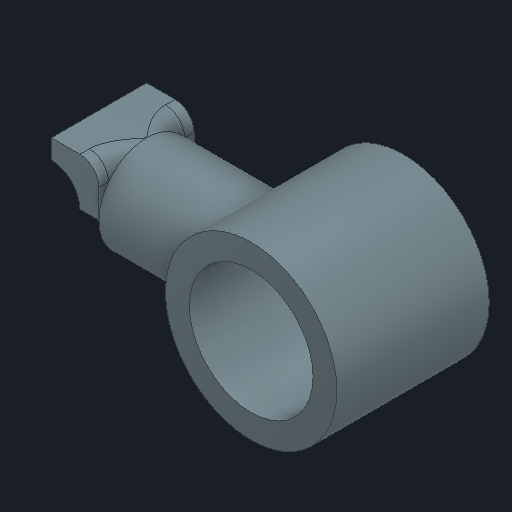
# Autodesk Inventor part: spojka_pol_stredne_koleso
Saved by Autodesk Inventor 2022 (Build 260153000, 153)
## iProperties
Created: 2021-12-17
Part Number: spojka_pol_stredne_koleso
Material: Lead
Document SubType Name: Modeling
Designer: MatusBarany
Density: 11.34 g/cm^3
Appearance: Lead
Author: MatusBarany
Autodesk Inventor part; units mm, degrees
ref_plane "XZ Plane" through (0, 0, 0) normal (0, 1, 0) x (-1, 0, 0)
sketch "Sketch1" plane through (0, 0, 0) normal (0, 0, 1) x (1, 0, 0)
  circle A0 centre (0, 0) radius 9
  circle A1 centre (0, 0) radius 6.5
  dimension "d0" = 13
  dimension "d1" = 18
  constraints: 2 centre point, 2 coincident
  measures "d0" diameter of A1
  measures "d1" diameter of A0
extrude "Extrusion1" add sketch "Sketch1" along normal blind 16
ref_plane "Work Plane2" through (-9, 0, 0) normal (1, 0, 0) x (0, 1, 0)
ref_plane "Work Plane1" through (0, 0, 0) normal (1, 0, 0) x (0, 1, 0)
sketch "Sketch2" plane through (-9, 0, 0) normal (1, 0, 0) x (0, 1, 0)
  line L0 (9, 0) -> (-9, 0) projected
  line L1 (9, 16) -> (-9, 16) projected
  line L2 (0, 0) -> (0, 16) construction
  circle A0 centre (0, 8) radius 5
  dimension "d6" = 10
  constraints: 2 end point, 2 midpoint, 1 centre point
  measures "d6" diameter of A0
extrude "Extrusion2" cut sketch "Sketch2" along normal blind 2
sketch "Sketch3" plane through (-7, 0, 8) normal (-1, 0, 0) x (0, 0, 1)
  circle A0 centre (0, 0) radius 5
  circle A1 centre (0, 0) radius 5 projected
  point P0 (-8, 0)
  dimension "d9" = 10
  constraints: 2 horizontal alignment, 1 centre point, 1 concentric
  measures "d9" diameter of A0
extrude "Extrusion3" add sketch "Sketch3" along normal blind 12
sketch "Sketch4" plane through (-19, 0, 8) normal (-1, 0, 0) x (0, 0, 1)
  circle A0 centre (0, 0) radius 5
  circle A1 centre (0, 0) radius 5 projected
  line L0 (-5, 0) -> (5, 0)
  point P0 (-8, 0)
  dimension "d12" = 10
  dimension "d13" = 10
  constraints: 2 end point, 2 point on circle, 1 centre point, 1 concentric, 1 horizontal
  measures "d12" diameter of A0
  measures "d13" distance of L0.start L0.end
extrude "Extrusion4" add sketch "Sketch4" along normal blind 5 contours L0 A0 picked at (1.2475, 1.1052)
ref_plane "Work Plane3" through (-7, 5, 8) normal (0, -1, 0) x (1, 0, 0)
sketch "Sketch7" plane through (-19, 0, 3) normal (0, -1, 0) x (1, 0, 0)
  line L0 (0, 10) -> (0, 0) projected
  line L1 (0, 10) -> (-5, 10) projected
  line L2 (-5, 0) -> (-5, 10) projected
  line L3 (0, 0) -> (-5, 0) projected
  point P0 (19, -3)
extrude "Extrusion6" add sketch "Sketch7" against normal blind 5
sketch "Sketch9" plane through (-19, 0, 3) normal (0, 0, -1) x (-1, 0, 0)
  line L0 (0, 0) -> (5, 0) projected
  line L1 (5, 0) -> (5, 5) projected
  line L2 (0, 5) -> (5, 5) projected
  line L3 (0, 0) -> (0, 5) projected
  circle A0 centre (5, 0) radius 3
  point P0 (-19, 0)
  point P1 (5, 3)
  point P2 (2, 0)
  dimension "d34" = 6
  constraints: 1 centre point, 1 coincident
  measures "d34" diameter of A0
extrude "Extrusion8" cut sketch "Sketch9" against normal through all contours A0 L1 L0 picked at (3.3172, 1.0574)
fillet "Fillet1" radius 2 2 edges at (-19, 5, 5.5) (-19, 5, 10.5)
body "Solid1"
